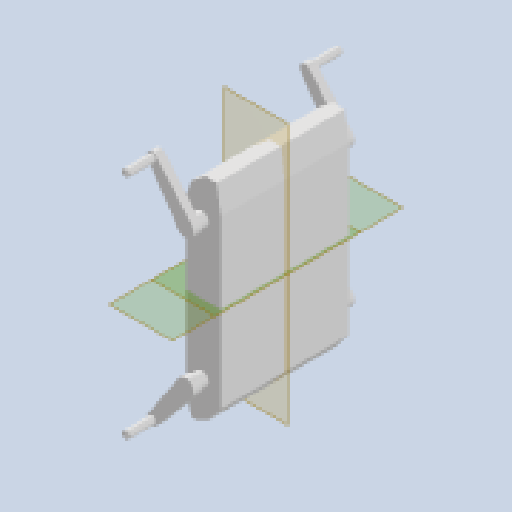
# Autodesk Inventor part: Body
Saved by Autodesk Inventor 2025 (Build 290162000, 162)
## iProperties
Created: 2025-12-16
Part Number: Body
Material: Типовые
Document SubType Name: Modeling
Designer: Artem Sannikov
Density: 1 g/cm^3
Appearance: По умолчанию
Author: Artem Sannikov
Autodesk Inventor part; units mm, degrees
ref_plane "YZ Plane" through (0, 0, 0) normal (1, 0, 0) x (0, 1, 0)
ref_plane "XZ Plane" through (0, 0, 0) normal (0, 1, 0) x (-1, 0, 0)
ref_plane "XY Plane" through (0, 0, 0) normal (0, 0, 1) x (1, 0, 0)
sketch "Эскиз1" plane through (0, 0, 0) normal (0, 0, 1) x (1, 0, 0)
  circle A0 centre (0, -10) radius 2.5 projected
  circle A1 centre (0, -10) radius 9.279
  point P0 (0, 0)
  constraints: 1 centre point, 1 coincident
extrude "Выдавливание1" add sketch "Эскиз1" along normal blind 64.5
sketch "Эскиз2" plane through (0, -10, 64.5) normal (0, 0, 1) x (1, 0, 0)
  circle A0 centre (0, 0) radius 2.5 projected
  circle A1 centre (0, 0) radius 12.9294
  circle A2 centre (81.1378, 108.3583) radius 20.7499
  line L0 (63.8374, 119.8151) -> (-10.7799, 7.1388)
  line L1 (97.0011, 94.9824) -> (9.8845, -8.3346)
  point P0 (0, 10)
  constraints: 4 end point, 4 point on circle, 4 tangent, 2 centre point, 1 coincident
extrude "Выдавливание2" add sketch "Эскиз2" along normal blind 20 contours A0 | A1 | A1 L0 A2 L1 | A2
sketch "Эскиз3" plane through (0, -10, 84.5) normal (0, 0, 1) x (1, 0, 0)
  point P0 (0, 10)
sketch "Эскиз4" plane through (0, -10, 84.5) normal (0, 0, 1) x (1, 0, 0)
  arc A0 (97.0011, 94.9824) -> (63.8374, 119.8151) centre (81.1378, 108.3583) ccw projected
  circle A1 centre (81.1378, 108.3583) radius 16.6702
  point P0 (0, 10)
  constraints: 1 centre point, 1 coincident
extrude "Выдавливание3" add sketch "Эскиз4" along normal blind 20
sketch "Эскиз5" plane through (81.1378, 98.3583, 104.5) normal (0, 0, 1) x (1, 0, 0)
  line L0 (46.5378, -41.7639) -> (-39.7786, -41.7639)
  line L1 (-39.7786, -41.7639) -> (-39.7786, 365.0024)
  line L2 (-39.7786, 365.0024) -> (46.5378, 365.0024)
  line L3 (46.5378, 365.0024) -> (46.5378, -41.7639)
  point P0 (-81.1378, -98.3583)
  constraints: 8 end point, 2 parallel, 1 horizontal, 1 perpendicular
extrude "Выдавливание4" add sketch "Эскиз5" along normal blind 313.25
sketch "Эскиз6" plane through (81.1378, 98.3583, 417.75) normal (0, 0, 1) x (1, 0, 0)
  line L0 (-39.7786, -41.7639) -> (46.5378, -41.7639) projected
  line L1 (46.5378, -41.7639) -> (17.3449, -79.2781)
  line L2 (17.3449, -79.2781) -> (-10.0163, -94.0317)
  line L3 (-10.0163, -94.0317) -> (-26.3794, -94.0317)
  line L4 (-26.3794, -94.0317) -> (-39.7786, -41.7639)
  line L5 (46.5378, 365.0024) -> (-39.7786, 365.0024) projected
  line L6 (-39.7786, 365.0024) -> (-26.3794, 404.6554)
  line L7 (-26.3794, 404.6554) -> (8.7844, 432.1543)
  line L8 (8.7844, 432.1543) -> (36.9707, 432.1543)
  line L9 (36.9707, 432.1543) -> (46.5378, 365.0024)
  point P0 (-81.1378, -98.3583)
  constraints: 16 end point, 2 parallel
extrude "Выдавливание5" add sketch "Эскиз6" against normal up to surface (313.25 mm away)
ref_plane "РабПлоскость1" through (54.7584, 267.4196, 417.75) normal (0, -1, 0) x (1, 0, 0)
mirror "Зеркальное отражение1" about plane through (54.7584, 267.4196, 417.75) normal (0, -1, 0) of "Выдавливание1", "Выдавливание2", "Выдавливание3"
ref_plane "РабПлоскость2" through (81.1378, 98.3583, 261.125) normal (0, 0, 1) x (1, 0, 0)
mirror "Зеркальное отражение2" about plane through (81.1378, 98.3583, 261.125) normal (0, 0, 1) of "Выдавливание1", "Выдавливание2", "Выдавливание3", "Выдавливание4", "Выдавливание5", "Зеркальное отражение1"
ref_plane "РабПлоскость3" through (54.7584, 267.4196, 104.5) normal (0, 1, 0) x (1, 0, 0)
